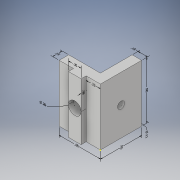
# Autodesk Inventor part: Part v4
Saved by Autodesk Inventor 2018 (Build 220112000, 112)
## iProperties
Created: 2019-12-09
Part Number: Part v4
Material: Generic
Document SubType Name: Modeling
Designer: AOFUser
Density: 1 g/cm^3
Appearance: Default
Author: AOFUser
Autodesk Inventor part; units mm, degrees
ref_plane "YZ Plane" through (0, 0, 0) normal (1, 0, 0) x (0, 1, 0)
ref_plane "XZ Plane" through (0, 0, 0) normal (0, 1, 0) x (-1, 0, 0)
ref_plane "XY Plane" through (0, 0, 0) normal (0, 0, 1) x (1, 0, 0)
sketch "Sketch1" plane through (0, 0, 0) normal (0, 1, 0) x (-1, 0, 0)
  line L0 (0, 0) -> (-16.51, 0)
  line L1 (-16.51, 0) -> (-16.51, -3.81)
  line L2 (-16.51, -3.81) -> (0, -3.81)
  line L3 (0, -3.81) -> (0, 0)
  line L4 (-16.51, 0) -> (-10.795, 0)
  line L5 (-10.795, 0) -> (-5.715, 0)
  line L6 (-5.715, 0) -> (-5.715, 2.032)
  line L7 (-5.715, 2.032) -> (-10.795, 2.032)
  line L8 (-10.795, 2.032) -> (-10.795, 0)
  line L9 (-16.51, 0) -> (-16.51, -16.51)
  line L10 (-16.51, -16.51) -> (-12.7, -16.51)
  line L11 (-12.7, -16.51) -> (-12.7, 0)
  dimension "d0" = 16.51
  dimension "d1" = 3.81
  dimension "d2" = 5.715
  dimension "d3" = 5.08
  dimension "d4" = 2.032
  dimension "d5" = 16.51
  dimension "d6" = 3.81
  constraints: 24 end point, 5 perpendicular, 3 parallel, 3 point on line, 1 horizontal, 1 vertical
  measures "d0" distance of L2.end L1.end
  measures "d1" distance of L1.end L0.end
  measures "d2" distance of L0.end L4.end
  measures "d3" distance of L4.end L5.end
  measures "d4" distance of L5.end L6.end
  measures "d5" distance of L0.end L9.end
  measures "d6" distance of L9.end L10.end
extrude "Extrusion1" add sketch "Sketch1" along normal blind 22.86
sketch "Sketch2" plane through (16.51, 0, 0) normal (1, 0, 0) x (0, 0, -1)
  point P0 (0, 0)
sketch "Sketch4" plane through (16.51, 0, 0) normal (1, 0, 0) x (0, 0, -1)
  line L0 (0, 0) -> (0, 22.86) projected
  line L1 (0, 11.43) -> (8.255, 11.43)
  dimension "d17" = 8.255
  constraints: 2 end point, 1 horizontal, 1 midpoint
  measures "d17" distance of L1.start L1.end
hole "Hole2" at (16.51, 11.43, -8.255) direction (-1, 0, 0) diameter 2.794 end through all
sketch "Sketch5" plane through (12.7, 0, -3.81) normal (0, 0, -1) x (-1, 0, 0)
  line L0 (0, 22.86) -> (12.7, 22.86) projected
  line L1 (12.7, 22.86) -> (4.445, 22.86)
  line L2 (4.445, 22.86) -> (4.445, 11.43)
  point P0 (12.7, 0)
  dimension "d46" = 8.255
  dimension "d47" = 11.43
  constraints: 4 end point, 1 perpendicular, 1 point on line
  measures "d46" distance of L0.end L1.end
  measures "d47" distance of L1.end L2.end
sketch "Sketch6" plane through (12.7, 0, -3.81) normal (0, 0, -1) x (-1, 0, 0)
  point P0 (12.7, 0)
hole "Hole3" at (8.255, 11.43, -3.81) direction (0, 0, 1) diameter 5.08 end through all
body "Solid1"
